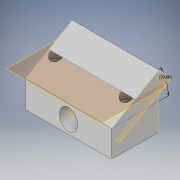
# Autodesk Inventor part: swallowMountV02
Saved by Autodesk Inventor 2019.4 (Build 234330000, 330)
## iProperties
Created: 2019-05-14
Part Number: swallowMountV02
Material: Generic
Document SubType Name: Modeling
Designer: steele
Density: 1 g/cm^3
Appearance: Default
Author: steele
Autodesk Inventor part; units mm, degrees
ref_plane "YZ Plane" through (0, 0, 0) normal (1, 0, 0) x (0, 1, 0)
sketch "Sketch2" plane through (0, 0, 0) normal (0, 0, 1) x (1, 0, 0)
  line L0 (0, 0) -> (69.85, 0)
  line L1 (69.85, 0) -> (69.85, 43.18)
  line L2 (69.85, 43.18) -> (0, 43.18)
  line L3 (0, 0) -> (0, 43.18) construction
  line L4 (0, 0) -> (-69.85, 0)
  line L5 (-69.85, 0) -> (-69.85, 43.18)
  line L6 (-69.85, 43.18) -> (0, 43.18)
  dimension "d2" = 69.85
  dimension "frontHeight" = 43.18
  constraints: 14 end point, 2 perpendicular, 2 symmetric about line, 1 horizontal, 1 parallel, 1 vertical
  measures "d2" distance of L0.start L0.end
  measures "frontHeight" distance of L0.end L1.end
ref_plane "Work Plane1" through (0, 0, -76.2) normal (0, 0, 1) x (1, 0, 0)
sketch "Sketch3" plane through (0, 0, -76.2) normal (0, 0, 1) x (1, 0, 0)
  line L0 (0, 0) -> (69.85, 0)
  line L1 (69.85, 0) -> (69.85, 87.1741)
  line L2 (69.85, 87.1741) -> (0, 87.1741)
  line L3 (0, 0) -> (0, 87.1741) construction
  line L4 (0, 0) -> (-69.85, 0)
  line L5 (-69.85, 0) -> (-69.85, 87.1741)
  line L6 (-69.85, 87.1741) -> (0, 87.1741)
  dimension "d5" = 69.85
  dimension "rearHeight" = 87.1741
  constraints: 14 end point, 2 perpendicular, 2 symmetric about line, 1 horizontal, 1 parallel, 1 vertical
  measures "d5" distance of L0.start L0.end
  measures "rearHeight" distance of L0.end L1.end
loft "Loft1" add profiles "Sketch2", "Sketch3"
sketch "Sketch4" plane through (69.85, 0, -76.2) normal (1, 0, 0) x (0, 0, -1)
  line L0 (-76.2, 43.18) -> (0, 87.1741) construction
  line L1 (-76.2, 43.18) -> (0, 43.18) construction
  line L2 (0, 0) -> (0, 87.1741) construction
  point P0 (-76.2, 0)
  dimension "d11" = 30
  constraints: 2 end point, 1 horizontal, 1 point on line
  measures "d11" angle of L0 L1
sketch "Sketch5" plane through (-69.85, 43.18, 0) normal (0, 0.866, 0.5) x (1, 0, 0)
  line L0 (0, 0) -> (0, 87.9882) construction
  line L1 (0, 43.9941) -> (139.7, 43.9941) construction
  line L2 (139.7, 0) -> (139.7, 87.9882) construction
  point P0 (69.85, -21.59)
  constraints: 2 end point, 2 midpoint
ref_plane "Work Plane2" through (-69.85, 65.177, -38.1) normal (0, -0.5, 0.866) x (1, 0, 0)
sketch "Sketch6" plane through (-69.85, 65.177, -38.1) normal (0, -0.5, 0.866) x (1, 0, 0)
  circle A0 centre (69.85, -19.05) radius 14.605
  line L0 (139.7, 0) -> (0, 0) projected
  point P0 (69.85, -37.395)
  dimension "holeDiameter" = 29.21
  dimension "centerLineForHole" = 19.05
  constraints: 1 centre point
  measures "holeDiameter" diameter of A0
  measures "centerLineForHole" distance from line of A0.centre L0
extrude "Extrusion1" cut sketch "Sketch6" along normal through all both and the other way through all
ref_plane "centerLineForHoleWork Plane" through (-69.85, 26.6822, -9.525) normal (0, 0.866, 0.5) x (1, 0, 0)
ref_plane "screwHoleWork Plane" through (69.85, 65.177, -38.1) normal (0, 1, 0) x (-1, 0, 0)
sketch "Sketch7" plane through (69.85, 65.177, -38.1) normal (0, 1, 0) x (-1, 0, 0)
  line L0 (0, -38.1) -> (139.7, -38.1) construction
  line L1 (69.85, -38.1) -> (69.85, 38.1) construction
  point P0 (127, 0)
  point P1 (12.7, 0)
  dimension "d18" = 57.15
  dimension "d19" = 57.15
  constraints: 2 end point, 1 midpoint, 1 vertical
  measures "d18" distance from line of point (127, 0) L1
  measures "d19" distance from line of point (12.7, 0) L1
hole "Hole1" at (-57.15, 65.177, -38.1) at (57.15, 65.177, -38.1) direction (0, -1, 0) diameter 7.1374 end through all counterbore diameter 19.05 counterbore depth 12.7 clearance for "Hex Head Bolt" size "1/4" standard "Ansi Unified Screw Threads"
equation "\"d2\" = 0.5 * width"
equation "\"d5\" = 0.5 * width"
equation "\"rearHeight\" = frontHeight + 0.57735 * depth"
equation "\"d18\" = holeDistanceFromCenter"
equation "\"d19\" = holeDistanceFromCenter"
equation "\"width\" = 139.7"
equation "\"d4\" = -depth"
equation "\"depth\" = 76.2"
equation "\"d17\" = -centerLineForHole"
equation "\"holeDistanceFromCenter\" = 57.15"
body "Solid1"
